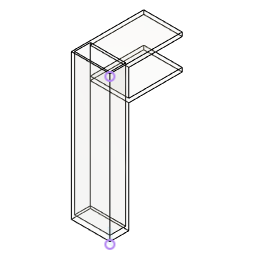
Craft Saw Desk Sheath v4 (Autodesk Fusion 360 design; units mm, degrees)
Autodesk Fusion 360 part; units mm, degrees
sketch "Sketch1" plane through (0, 0, 0) normal (0, 1, 0) x (1, 0, 0)
  line L0 (2.9948, -0.9169) -> (7.4948, -0.9169)
  line L1 (7.4948, -0.9169) -> (7.4948, -18.9169)
  line L2 (7.4948, -18.9169) -> (2.9948, -18.9169)
  line L3 (2.9948, -18.9169) -> (2.9948, -0.9169)
  dimension "d1" = 4.5
  dimension "d2" = 18
  constraint horizontal L0
  constraint vertical L1
  constraint horizontal L2
  constraint vertical L3
  measures "d1" distance of L0.start L0.end
  measures "d2" distance of L0.start L2.end
sketch "Sketch2" plane through (0, 0, 18.9169) normal (0, 0, 1) x (-1, 0, 0)
  line L0 (-2.9948, 0) -> (-7.4948, 0)
  line L1 (-7.4948, 0) -> (-7.4948, -2)
  line L2 (-7.4948, -2) -> (-2.9948, -2)
  line L3 (-2.9948, -2) -> (-2.9948, 0)
  line L4 (-7.4948, 0) -> (-2.9948, 0)
  line L5 (-2.9948, 0.5) -> (-7.4948, 0.5)
  line L6 (-2.9948, 0) -> (-3.4948, 0)
  line L7 (-3.4948, -2) -> (-2.9948, -2)
  line L8 (-2.9948, -2) -> (-2.9948, 0)
  line L9 (-2.9948, -2) -> (-7.4948, -2)
  line L10 (-7.4948, -2.5) -> (-2.9948, -2.5)
  line L11 (-7.4948, 0.5) -> (-7.9948, 0.5)
  line L12 (-7.9948, 0.5) -> (-7.9948, -2.5)
  line L13 (-7.9948, -2.5) -> (-7.4948, -2.5)
  line L14 (-2.9948, 0.5) -> (-2.4948, 0.5)
  line L15 (-2.4948, 0.5) -> (-2.4948, -2.5)
  line L16 (-2.4948, -2.5) -> (-2.9948, -2.5)
  dimension "d5" = 0.5
  dimension "d6" = 0.5
  dimension "d7" = 2
  dimension "d8" = 4.5
  dimension "d9" = 0.5
  dimension "d10" = 0.5
  dimension "d11" = 3
  dimension "d12" = 0.5
  dimension "d13" = 3
  constraint horizontal L4
  constraint horizontal L5
  constraint coincident L0.end L1.start
  constraint horizontal L6
  constraint horizontal L7
  constraint vertical L8
  constraint coincident L0.start L3.end
  constraint horizontal L9
  constraint horizontal L10
  constraint coincident L2.end L3.start
  constraint horizontal L11
  constraint vertical L12
  constraint horizontal L13
  constraint horizontal L14
  constraint vertical L15
  constraint horizontal L16
  measures "d5" distance of L0.end L5.end
  measures "d6" distance of L0.start L6.end
  measures "d7" distance of L0.start L2.end
  measures "d8" distance of L2.end L1.end
  measures "d9" distance of L2.end L10.end
  measures "d10" distance of L5.end L11.end
  measures "d11" distance of L5.end L10.start
  measures "d12" distance of L5.start L14.end
  measures "d13" distance of L5.start L10.end
extrude "Extrude2" add sketch "Sketch2" against normal blind 18
sketch "Sketch3" plane through (0, 0, 0.9169) normal (0, 0, -1) x (1, 0, 0)
  line L0 (2.9948, 0) -> (7.4948, 0)
  line L1 (7.4948, 0) -> (7.4948, -2)
  line L2 (7.4948, -2) -> (2.9948, -2)
  line L3 (2.9948, -2) -> (2.9948, 0)
  line L4 (7.9948, 0.5) -> (2.4948, 0.5)
  line L5 (2.4948, 0.5) -> (2.4948, -2.5)
  line L6 (2.4948, -2.5) -> (7.9948, -2.5)
  line L7 (7.9948, -2.5) -> (7.9948, 0.5)
  line L8 (7.9948, 0.5) -> (2.4948, 0.5)
  line L9 (2.4948, 0.5) -> (2.4948, -2.5)
  line L10 (2.4948, -2.5) -> (7.9948, -2.5)
  line L11 (7.9948, -2.5) -> (7.9948, 0.5)
  constraint horizontal L8
  constraint vertical L9
  constraint horizontal L10
  constraint vertical L11
  constraint coincident L5.end L6.start
  constraint coincident L4.start L7.end
extrude "Extrude3" add sketch "Sketch3" along normal blind 0.5 contours L0 L1 L2 L3 | L4 L5 L6 L7 L8 L9 L10 L11
sketch "Sketch4" plane through (0, 2.5, 0) normal (0, 1, 0) x (-1, 0, 0)
  line L0 (-2.4948, 18.9169) -> (-7.9948, 18.9169)
  line L1 (-7.9948, 18.9169) -> (-7.9948, 0.4169)
  line L2 (-7.9948, 0.4169) -> (-2.4948, 0.4169)
  line L3 (-2.4948, 0.4169) -> (-2.4948, 18.9169)
scale "Scale1" factor 10 about (7.9948, -0.5, 18.9169) bodies 1
sketch "Sketch5" plane through (0, 29.5, 0) normal (0, 1, 0) x (-1, 0, 0)
  line L0 (47.0052, 18.9169) -> (-7.9948, 18.9169)
  line L1 (-7.9948, 18.9169) -> (-7.9948, -166.0831)
  line L2 (-7.9948, -166.0831) -> (47.0052, -166.0831)
  line L3 (47.0052, -166.0831) -> (47.0052, 18.9169)
  line L4 (-7.9948, 18.9169) -> (47.0052, 18.9169)
  line L5 (47.0052, 18.9169) -> (47.0052, 13.9169)
  line L6 (47.0052, 13.9169) -> (-7.9948, 13.9169)
  line L7 (-7.9948, 13.9169) -> (-7.9948, 18.9169)
  line L8 (-7.9948, -20.0831) -> (47.0052, -20.0831)
  line L9 (47.0052, -20.0831) -> (47.0052, -25.0831)
  line L10 (47.0052, -25.0831) -> (-7.9948, -25.0831)
  line L11 (-7.9948, -25.0831) -> (-7.9948, -20.0831)
  dimension "d19" = 5
  dimension "d20" = 34
  dimension "d21" = 5
  constraint horizontal L4
  constraint vertical L5
  constraint horizontal L6
  constraint vertical L7
  constraint coincident L0.end L1.start
  constraint horizontal L8
  constraint vertical L9
  constraint horizontal L10
  constraint vertical L11
  measures "d19" distance of L0.end L6.end
  measures "d20" distance of L6.end L8.start
  measures "d21" distance of L8.start L10.end
extrude "Extrude4" add sketch "Sketch5" along normal blind 65 contours L0 L1 L3 L4 L5 L6 L7 | L1 L3 L8 L9 L10 L11
move_body "Move1" bodies 1 to x (1, 0, 0) y (0, 1, 0) z (0, 0, 1) at (0, 0, 170)
sketch "Sketch6" plane through (7.9948, 0, 0) normal (1, 0, 0) x (0, 1, 0)
  line L0 (94.5, 188.9169) -> (-0.5, 188.9169)
  line L1 (-0.5, 3.9169) -> (29.5, 3.9169)
  line L2 (29.5, 3.9169) -> (29.5, 144.9169)
  line L3 (29.5, 144.9169) -> (94.5, 144.9169)
  line L4 (94.5, 144.9169) -> (94.5, 149.9169)
  line L5 (94.5, 149.9169) -> (29.5, 149.9169)
  line L6 (29.5, 149.9169) -> (29.5, 183.9169)
  line L7 (29.5, 183.9169) -> (94.5, 183.9169)
  line L8 (94.5, 183.9169) -> (94.5, 188.9169)
sketch "Sketch7" plane through (-47.0052, 0, 0) normal (-1, 0, 0) x (0, -1, 0)
  line L0 (0.5, 188.9169) -> (-94.5, 188.9169)
  line L1 (-94.5, 188.9169) -> (-94.5, 183.9169)
  line L2 (-94.5, 183.9169) -> (-29.5, 183.9169)
  line L3 (-29.5, 183.9169) -> (-29.5, 149.9169)
  line L4 (-29.5, 149.9169) -> (-94.5, 149.9169)
  line L5 (-94.5, 149.9169) -> (-94.5, 144.9169)
  line L6 (-94.5, 144.9169) -> (-29.5, 144.9169)
  line L7 (-29.5, 144.9169) -> (-29.5, 3.9169)
  line L8 (-29.5, 3.9169) -> (0.5, 3.9169)
  line L9 (0.5, 3.9169) -> (0.5, 188.9169)
extrude "Extrude5" cut 2 faces at (-10.3385, 29.5, 172.5836) (-10.3385, 29.5, 50.9169) along direction (0, -1, 0) blind 3
extrude "Extrude6" cut 1 faces at (-10.3385, -0.5, 127.2503) along direction (0, 1, 0) blind 3
extrude "Extrude7" cut sketch "Sketch7" against normal blind 3
extrude "Extrude8" cut 1 faces at (7.9948, 10.5, 112.5836) along direction (-1, 0, 0) blind 3
